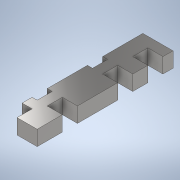
# Autodesk Inventor part: SujeciónSoportes
Saved by Autodesk Inventor 2020.2 (Build 242310000, 310)
## iProperties
Created: 2020-03-18
Part Number: SujeciónSoportes
Material: Steel, Alloy
Document SubType Name: Modeling
Designer: ARQ SEVILLA R
Density: 7.73 g/cm^3
Appearance: Semi-Polished
Author: ARQ SEVILLA R
Autodesk Inventor part; units mm, degrees
ref_plane "YZ Plane" through (0, 0, 0) normal (1, 0, 0) x (0, 1, 0)
ref_plane "XZ Plane" through (0, 0, 0) normal (0, 1, 0) x (-1, 0, 0)
ref_plane "XY Plane" through (0, 0, 0) normal (0, 0, 1) x (1, 0, 0)
sketch "Sketch1" plane through (0, 0, 0) normal (0, 1, 0) x (-1, 0, 0)
  line L0 (0, 0) -> (4, 0)
  line L1 (4, 0) -> (4, -3)
  line L2 (4, -3) -> (6, -3)
  line L3 (6, -3) -> (6, -27)
  line L4 (6, -27) -> (0, -27)
  line L5 (0, 0) -> (0, -5)
  line L6 (0, -5) -> (3, -5)
  line L7 (3, -5) -> (3, -8)
  line L8 (3, -8) -> (0, -8)
  line L9 (0, -8) -> (0, -16)
  line L10 (0, -16) -> (3, -16)
  line L11 (3, -16) -> (3, -19)
  line L12 (3, -19) -> (0, -19)
  line L13 (0, -19) -> (0, -22)
  line L14 (0, -22) -> (3, -22)
  line L15 (3, -22) -> (3, -25)
  line L16 (3, -25) -> (0, -25)
  line L17 (0, -25) -> (0, -27)
  dimension "d0" = 4
  dimension "d1" = 3
  dimension "d2" = 2
  dimension "d3" = 24
  dimension "d4" = 5
  dimension "d6" = 3
  dimension "d7" = 8
  dimension "d8" = 3
  dimension "d9" = 3
  dimension "d10" = 3
  dimension "d11" = 3
  dimension "d12" = 3
  dimension "d13" = 3
  constraints: 36 end point, 6 perpendicular, 2 point on line, 1 horizontal
  measures "d0" distance of L0.start L0.end
  measures "d1" distance of L0.end L1.end
  measures "d2" distance of L1.end L2.end
  measures "d3" distance of L2.end L3.end
  measures "d4" distance of L0.start L5.end
  measures "d6" distance of L6.end L7.end
  measures "d7" distance of L8.end L9.end
  measures "d8" distance of L9.end L10.end
  measures "d9" distance of L10.end L11.end
  measures "d10" distance of L12.end L13.end
  measures "d11" distance of L13.end L14.end
  measures "d12" distance of L14.end L15.end
  measures "d13" distance of L15.end L16.end
extrude "Extrusion1" add sketch "Sketch1" along normal blind 3
sketch "Sketch2" plane through (0, 0, 0) normal (0, -1, 0) x (1, 0, 0)
  line L0 (-3, -16) -> (-3, -19) projected
  line L1 (-6, -27) -> (-6, -3) projected
  line L2 (-6, -16) -> (-5, -16)
  line L3 (-5, -16) -> (-5, -19)
  line L4 (-3, -19) -> (0, -19) projected
  line L5 (-5, -19) -> (-6, -19)
  line L6 (-3, -5) -> (-3, -8) projected
  line L7 (-5, -8) -> (-6, -8)
  line L8 (-5, -8) -> (-5, -5)
  line L9 (-5, -5) -> (-6, -5)
  point P0 (0, 0)
  dimension "d16" = 1
  constraints: 12 end point, 3 perpendicular, 3 point on line, 1 horizontal, 1 vertical
  measures "d16" distance of L2.start L2.end
extrude "Extrusion2" cut sketch "Sketch2" against normal up to surface (3 mm away)
body "Solid1"
